Autodesk Fusion 360 part; units mm, degrees
(part 2 of 2)
sketch "Sketch26" plane through (0, 0, -20) normal (0, 0, -1) x (1, 0, 0)
  line L0 (49.5, -31.5) -> (-49.5, 31.5) construction
  line L1 (-49.5, -31.5) -> (49.5, 31.5) construction
  line L2 (-46.9725, 28.9725) -> (-52.0275, 28.9725)
  line L3 (-52.0275, 28.9725) -> (-52.0275, 34.0275)
  line L4 (-52.0275, 34.0275) -> (-46.9725, 34.0275)
  line L5 (-46.9725, 34.0275) -> (-46.9725, 28.9725)
  line L6 (-46.9725, 28.9725) -> (-52.0275, 34.0275) construction
  line L7 (-52.0275, 28.9725) -> (-46.9725, 34.0275) construction
  line L8 (-37.9725, 28.9725) -> (-43.0275, 28.9725)
  line L9 (-43.0275, 28.9725) -> (-43.0275, 34.0275)
  line L10 (-43.0275, 34.0275) -> (-37.9725, 34.0275)
  line L11 (-37.9725, 34.0275) -> (-37.9725, 28.9725)
  line L12 (-28.9725, 28.9725) -> (-34.0275, 28.9725)
  line L13 (-34.0275, 28.9725) -> (-34.0275, 34.0275)
  line L14 (-34.0275, 34.0275) -> (-28.9725, 34.0275)
  line L15 (-28.9725, 34.0275) -> (-28.9725, 28.9725)
  line L16 (-19.9725, 28.9725) -> (-25.0275, 28.9725)
  line L17 (-25.0275, 28.9725) -> (-25.0275, 34.0275)
  line L18 (-25.0275, 34.0275) -> (-19.9725, 34.0275)
  line L19 (-19.9725, 34.0275) -> (-19.9725, 28.9725)
  line L20 (-10.9725, 28.9725) -> (-16.0275, 28.9725)
  line L21 (-16.0275, 28.9725) -> (-16.0275, 34.0275)
  line L22 (-16.0275, 34.0275) -> (-10.9725, 34.0275)
  line L23 (-10.9725, 34.0275) -> (-10.9725, 28.9725)
  line L24 (-1.9725, 28.9725) -> (-7.0275, 28.9725)
  line L25 (-7.0275, 28.9725) -> (-7.0275, 34.0275)
  line L26 (-7.0275, 34.0275) -> (-1.9725, 34.0275)
  line L27 (-1.9725, 34.0275) -> (-1.9725, 28.9725)
  line L28 (7.0275, 28.9725) -> (1.9725, 28.9725)
  line L29 (1.9725, 28.9725) -> (1.9725, 34.0275)
  line L30 (1.9725, 34.0275) -> (7.0275, 34.0275)
  line L31 (7.0275, 34.0275) -> (7.0275, 28.9725)
  line L32 (16.0275, 28.9725) -> (10.9725, 28.9725)
  line L33 (10.9725, 28.9725) -> (10.9725, 34.0275)
  line L34 (10.9725, 34.0275) -> (16.0275, 34.0275)
  line L35 (16.0275, 34.0275) -> (16.0275, 28.9725)
  line L36 (25.0275, 28.9725) -> (19.9725, 28.9725)
  line L37 (19.9725, 28.9725) -> (19.9725, 34.0275)
  line L38 (19.9725, 34.0275) -> (25.0275, 34.0275)
  line L39 (25.0275, 34.0275) -> (25.0275, 28.9725)
  line L40 (34.0275, 28.9725) -> (28.9725, 28.9725)
  line L41 (28.9725, 28.9725) -> (28.9725, 34.0275)
  line L42 (28.9725, 34.0275) -> (34.0275, 34.0275)
  line L43 (34.0275, 34.0275) -> (34.0275, 28.9725)
  line L44 (43.0275, 28.9725) -> (37.9725, 28.9725)
  line L45 (37.9725, 28.9725) -> (37.9725, 34.0275)
  line L46 (37.9725, 34.0275) -> (43.0275, 34.0275)
  line L47 (43.0275, 34.0275) -> (43.0275, 28.9725)
  line L48 (52.0275, 28.9725) -> (46.9725, 28.9725)
  line L49 (46.9725, 28.9725) -> (46.9725, 34.0275)
  line L50 (46.9725, 34.0275) -> (52.0275, 34.0275)
  line L51 (52.0275, 34.0275) -> (52.0275, 28.9725)
  line L52 (-46.9725, 19.9725) -> (-52.0275, 19.9725)
  line L53 (-52.0275, 19.9725) -> (-52.0275, 25.0275)
  line L54 (-52.0275, 25.0275) -> (-46.9725, 25.0275)
  line L55 (-46.9725, 25.0275) -> (-46.9725, 19.9725)
  line L56 (-37.9725, 19.9725) -> (-43.0275, 19.9725)
  line L57 (-43.0275, 19.9725) -> (-43.0275, 25.0275)
  line L58 (-43.0275, 25.0275) -> (-37.9725, 25.0275)
  line L59 (-37.9725, 25.0275) -> (-37.9725, 19.9725)
  line L60 (-28.9725, 19.9725) -> (-34.0275, 19.9725)
  line L61 (-34.0275, 19.9725) -> (-34.0275, 25.0275)
  line L62 (-34.0275, 25.0275) -> (-28.9725, 25.0275)
  line L63 (-28.9725, 25.0275) -> (-28.9725, 19.9725)
  line L64 (-19.9725, 19.9725) -> (-25.0275, 19.9725)
  line L65 (-25.0275, 19.9725) -> (-25.0275, 25.0275)
  line L66 (-25.0275, 25.0275) -> (-19.9725, 25.0275)
  line L67 (-19.9725, 25.0275) -> (-19.9725, 19.9725)
  line L68 (-10.9725, 19.9725) -> (-16.0275, 19.9725)
  line L69 (-16.0275, 19.9725) -> (-16.0275, 25.0275)
  line L70 (-16.0275, 25.0275) -> (-10.9725, 25.0275)
  line L71 (-10.9725, 25.0275) -> (-10.9725, 19.9725)
  line L72 (-1.9725, 19.9725) -> (-7.0275, 19.9725)
  line L73 (-7.0275, 19.9725) -> (-7.0275, 25.0275)
  line L74 (-7.0275, 25.0275) -> (-1.9725, 25.0275)
  line L75 (-1.9725, 25.0275) -> (-1.9725, 19.9725)
  line L76 (7.0275, 19.9725) -> (1.9725, 19.9725)
  line L77 (1.9725, 19.9725) -> (1.9725, 25.0275)
  line L78 (1.9725, 25.0275) -> (7.0275, 25.0275)
  line L79 (7.0275, 25.0275) -> (7.0275, 19.9725)
  line L80 (16.0275, 19.9725) -> (10.9725, 19.9725)
  line L81 (10.9725, 19.9725) -> (10.9725, 25.0275)
  line L82 (10.9725, 25.0275) -> (16.0275, 25.0275)
  line L83 (16.0275, 25.0275) -> (16.0275, 19.9725)
  line L84 (25.0275, 19.9725) -> (19.9725, 19.9725)
  line L85 (19.9725, 19.9725) -> (19.9725, 25.0275)
  line L86 (19.9725, 25.0275) -> (25.0275, 25.0275)
  line L87 (25.0275, 25.0275) -> (25.0275, 19.9725)
  line L88 (34.0275, 19.9725) -> (28.9725, 19.9725)
  line L89 (28.9725, 19.9725) -> (28.9725, 25.0275)
  line L90 (28.9725, 25.0275) -> (34.0275, 25.0275)
  line L91 (34.0275, 25.0275) -> (34.0275, 19.9725)
  line L92 (43.0275, 19.9725) -> (37.9725, 19.9725)
  line L93 (37.9725, 19.9725) -> (37.9725, 25.0275)
  line L94 (37.9725, 25.0275) -> (43.0275, 25.0275)
  line L95 (43.0275, 25.0275) -> (43.0275, 19.9725)
  line L96 (52.0275, 19.9725) -> (46.9725, 19.9725)
  line L97 (46.9725, 19.9725) -> (46.9725, 25.0275)
  line L98 (46.9725, 25.0275) -> (52.0275, 25.0275)
  line L99 (52.0275, 25.0275) -> (52.0275, 19.9725)
  line L100 (-46.9725, 10.9725) -> (-52.0275, 10.9725)
  line L101 (-52.0275, 10.9725) -> (-52.0275, 16.0275)
  line L102 (-52.0275, 16.0275) -> (-46.9725, 16.0275)
  line L103 (-46.9725, 16.0275) -> (-46.9725, 10.9725)
  line L104 (-37.9725, 10.9725) -> (-43.0275, 10.9725)
  line L105 (-43.0275, 10.9725) -> (-43.0275, 16.0275)
  line L106 (-43.0275, 16.0275) -> (-37.9725, 16.0275)
  line L107 (-37.9725, 16.0275) -> (-37.9725, 10.9725)
  line L108 (-28.9725, 10.9725) -> (-34.0275, 10.9725)
  line L109 (-34.0275, 10.9725) -> (-34.0275, 16.0275)
  line L110 (-34.0275, 16.0275) -> (-28.9725, 16.0275)
  line L111 (-28.9725, 16.0275) -> (-28.9725, 10.9725)
  line L112 (-19.9725, 10.9725) -> (-25.0275, 10.9725)
  line L113 (-25.0275, 10.9725) -> (-25.0275, 16.0275)
  line L114 (-25.0275, 16.0275) -> (-19.9725, 16.0275)
  line L115 (-19.9725, 16.0275) -> (-19.9725, 10.9725)
  line L116 (-10.9725, 10.9725) -> (-16.0275, 10.9725)
  line L117 (-16.0275, 10.9725) -> (-16.0275, 16.0275)
  line L118 (-16.0275, 16.0275) -> (-10.9725, 16.0275)
  line L119 (-10.9725, 16.0275) -> (-10.9725, 10.9725)
  line L120 (-1.9725, 10.9725) -> (-7.0275, 10.9725)
  line L121 (-7.0275, 10.9725) -> (-7.0275, 16.0275)
  line L122 (-7.0275, 16.0275) -> (-1.9725, 16.0275)
  line L123 (-1.9725, 16.0275) -> (-1.9725, 10.9725)
  line L124 (7.0275, 10.9725) -> (1.9725, 10.9725)
  line L125 (1.9725, 10.9725) -> (1.9725, 16.0275)
  line L126 (1.9725, 16.0275) -> (7.0275, 16.0275)
  line L127 (7.0275, 16.0275) -> (7.0275, 10.9725)
  line L128 (16.0275, 10.9725) -> (10.9725, 10.9725)
  line L129 (10.9725, 10.9725) -> (10.9725, 16.0275)
  line L130 (10.9725, 16.0275) -> (16.0275, 16.0275)
  line L131 (16.0275, 16.0275) -> (16.0275, 10.9725)
  line L132 (25.0275, 10.9725) -> (19.9725, 10.9725)
  line L133 (19.9725, 10.9725) -> (19.9725, 16.0275)
  line L134 (19.9725, 16.0275) -> (25.0275, 16.0275)
  line L135 (25.0275, 16.0275) -> (25.0275, 10.9725)
  line L136 (34.0275, 10.9725) -> (28.9725, 10.9725)
  line L137 (28.9725, 10.9725) -> (28.9725, 16.0275)
  line L138 (28.9725, 16.0275) -> (34.0275, 16.0275)
  line L139 (34.0275, 16.0275) -> (34.0275, 10.9725)
  line L140 (43.0275, 10.9725) -> (37.9725, 10.9725)
  line L141 (37.9725, 10.9725) -> (37.9725, 16.0275)
  line L142 (37.9725, 16.0275) -> (43.0275, 16.0275)
  line L143 (43.0275, 16.0275) -> (43.0275, 10.9725)
  line L144 (52.0275, 10.9725) -> (46.9725, 10.9725)
  line L145 (46.9725, 10.9725) -> (46.9725, 16.0275)
  line L146 (46.9725, 16.0275) -> (52.0275, 16.0275)
  line L147 (52.0275, 16.0275) -> (52.0275, 10.9725)
  line L148 (-46.9725, 1.9725) -> (-52.0275, 1.9725)
  line L149 (-52.0275, 1.9725) -> (-52.0275, 7.0275)
  line L150 (-52.0275, 7.0275) -> (-46.9725, 7.0275)
  line L151 (-46.9725, 7.0275) -> (-46.9725, 1.9725)
  line L152 (-37.9725, 1.9725) -> (-43.0275, 1.9725)
  line L153 (-43.0275, 1.9725) -> (-43.0275, 7.0275)
  line L154 (-43.0275, 7.0275) -> (-37.9725, 7.0275)
  line L155 (-37.9725, 7.0275) -> (-37.9725, 1.9725)
  line L156 (-28.9725, 1.9725) -> (-34.0275, 1.9725)
  line L157 (-34.0275, 1.9725) -> (-34.0275, 7.0275)
  line L158 (-34.0275, 7.0275) -> (-28.9725, 7.0275)
  line L159 (-28.9725, 7.0275) -> (-28.9725, 1.9725)
  line L160 (-19.9725, 1.9725) -> (-25.0275, 1.9725)
  line L161 (-25.0275, 1.9725) -> (-25.0275, 7.0275)
  line L162 (-25.0275, 7.0275) -> (-19.9725, 7.0275)
  line L163 (-19.9725, 7.0275) -> (-19.9725, 1.9725)
  line L164 (-10.9725, 1.9725) -> (-16.0275, 1.9725)
  line L165 (-16.0275, 1.9725) -> (-16.0275, 7.0275)
  line L166 (-16.0275, 7.0275) -> (-10.9725, 7.0275)
  line L167 (-10.9725, 7.0275) -> (-10.9725, 1.9725)
  line L168 (-1.9725, 1.9725) -> (-7.0275, 1.9725)
  line L169 (-7.0275, 1.9725) -> (-7.0275, 7.0275)
  line L170 (-7.0275, 7.0275) -> (-1.9725, 7.0275)
  line L171 (-1.9725, 7.0275) -> (-1.9725, 1.9725)
  line L172 (7.0275, 1.9725) -> (1.9725, 1.9725)
  line L173 (1.9725, 1.9725) -> (1.9725, 7.0275)
  line L174 (1.9725, 7.0275) -> (7.0275, 7.0275)
  line L175 (7.0275, 7.0275) -> (7.0275, 1.9725)
  line L176 (16.0275, 1.9725) -> (10.9725, 1.9725)
  line L177 (10.9725, 1.9725) -> (10.9725, 7.0275)
  line L178 (10.9725, 7.0275) -> (16.0275, 7.0275)
  line L179 (16.0275, 7.0275) -> (16.0275, 1.9725)
  line L180 (25.0275, 1.9725) -> (19.9725, 1.9725)
  line L181 (19.9725, 1.9725) -> (19.9725, 7.0275)
  line L182 (19.9725, 7.0275) -> (25.0275, 7.0275)
  line L183 (25.0275, 7.0275) -> (25.0275, 1.9725)
  line L184 (34.0275, 1.9725) -> (28.9725, 1.9725)
  line L185 (28.9725, 1.9725) -> (28.9725, 7.0275)
  line L186 (28.9725, 7.0275) -> (34.0275, 7.0275)
  line L187 (34.0275, 7.0275) -> (34.0275, 1.9725)
  line L188 (43.0275, 1.9725) -> (37.9725, 1.9725)
  line L189 (37.9725, 1.9725) -> (37.9725, 7.0275)
  line L190 (37.9725, 7.0275) -> (43.0275, 7.0275)
  line L191 (43.0275, 7.0275) -> (43.0275, 1.9725)
  line L192 (52.0275, 1.9725) -> (46.9725, 1.9725)
  line L193 (46.9725, 1.9725) -> (46.9725, 7.0275)
  line L194 (46.9725, 7.0275) -> (52.0275, 7.0275)
  line L195 (52.0275, 7.0275) -> (52.0275, 1.9725)
  line L196 (-46.9725, -7.0275) -> (-52.0275, -7.0275)
  line L197 (-52.0275, -7.0275) -> (-52.0275, -1.9725)
  line L198 (-52.0275, -1.9725) -> (-46.9725, -1.9725)
  line L199 (-46.9725, -1.9725) -> (-46.9725, -7.0275)
  line L200 (-37.9725, -7.0275) -> (-43.0275, -7.0275)
  line L201 (-43.0275, -7.0275) -> (-43.0275, -1.9725)
  line L202 (-43.0275, -1.9725) -> (-37.9725, -1.9725)
  line L203 (-37.9725, -1.9725) -> (-37.9725, -7.0275)
  line L204 (-28.9725, -7.0275) -> (-34.0275, -7.0275)
  line L205 (-34.0275, -7.0275) -> (-34.0275, -1.9725)
  line L206 (-34.0275, -1.9725) -> (-28.9725, -1.9725)
  line L207 (-28.9725, -1.9725) -> (-28.9725, -7.0275)
  line L208 (-19.9725, -7.0275) -> (-25.0275, -7.0275)
  line L209 (-25.0275, -7.0275) -> (-25.0275, -1.9725)
  line L210 (-25.0275, -1.9725) -> (-19.9725, -1.9725)
  line L211 (-19.9725, -1.9725) -> (-19.9725, -7.0275)
  line L212 (-10.9725, -7.0275) -> (-16.0275, -7.0275)
  line L213 (-16.0275, -7.0275) -> (-16.0275, -1.9725)
  line L214 (-16.0275, -1.9725) -> (-10.9725, -1.9725)
  line L215 (-10.9725, -1.9725) -> (-10.9725, -7.0275)
  line L216 (-1.9725, -7.0275) -> (-7.0275, -7.0275)
  line L217 (-7.0275, -7.0275) -> (-7.0275, -1.9725)
  line L218 (-7.0275, -1.9725) -> (-1.9725, -1.9725)
  line L219 (-1.9725, -1.9725) -> (-1.9725, -7.0275)
  line L220 (7.0275, -7.0275) -> (1.9725, -7.0275)
  line L221 (1.9725, -7.0275) -> (1.9725, -1.9725)
  line L222 (1.9725, -1.9725) -> (7.0275, -1.9725)
  line L223 (7.0275, -1.9725) -> (7.0275, -7.0275)
  line L224 (16.0275, -7.0275) -> (10.9725, -7.0275)
  line L225 (10.9725, -7.0275) -> (10.9725, -1.9725)
  line L226 (10.9725, -1.9725) -> (16.0275, -1.9725)
  line L227 (16.0275, -1.9725) -> (16.0275, -7.0275)
  line L228 (25.0275, -7.0275) -> (19.9725, -7.0275)
  line L229 (19.9725, -7.0275) -> (19.9725, -1.9725)
  line L230 (19.9725, -1.9725) -> (25.0275, -1.9725)
  line L231 (25.0275, -1.9725) -> (25.0275, -7.0275)
  line L232 (34.0275, -7.0275) -> (28.9725, -7.0275)
  line L233 (28.9725, -7.0275) -> (28.9725, -1.9725)
  line L234 (28.9725, -1.9725) -> (34.0275, -1.9725)
  line L235 (34.0275, -1.9725) -> (34.0275, -7.0275)
  line L236 (43.0275, -7.0275) -> (37.9725, -7.0275)
  line L237 (37.9725, -7.0275) -> (37.9725, -1.9725)
  line L238 (37.9725, -1.9725) -> (43.0275, -1.9725)
  line L239 (43.0275, -1.9725) -> (43.0275, -7.0275)
  line L240 (52.0275, -7.0275) -> (46.9725, -7.0275)
  line L241 (46.9725, -7.0275) -> (46.9725, -1.9725)
  line L242 (46.9725, -1.9725) -> (52.0275, -1.9725)
  line L243 (52.0275, -1.9725) -> (52.0275, -7.0275)
  line L244 (-46.9725, -16.0275) -> (-52.0275, -16.0275)
  line L245 (-52.0275, -16.0275) -> (-52.0275, -10.9725)
  line L246 (-52.0275, -10.9725) -> (-46.9725, -10.9725)
  line L247 (-46.9725, -10.9725) -> (-46.9725, -16.0275)
  line L248 (-37.9725, -16.0275) -> (-43.0275, -16.0275)
  line L249 (-43.0275, -16.0275) -> (-43.0275, -10.9725)
  line L250 (-43.0275, -10.9725) -> (-37.9725, -10.9725)
  line L251 (-37.9725, -10.9725) -> (-37.9725, -16.0275)
  line L252 (-28.9725, -16.0275) -> (-34.0275, -16.0275)
  line L253 (-34.0275, -16.0275) -> (-34.0275, -10.9725)
  line L254 (-34.0275, -10.9725) -> (-28.9725, -10.9725)
  line L255 (-28.9725, -10.9725) -> (-28.9725, -16.0275)
  line L256 (-19.9725, -16.0275) -> (-25.0275, -16.0275)
  line L257 (-25.0275, -16.0275) -> (-25.0275, -10.9725)
  line L258 (-25.0275, -10.9725) -> (-19.9725, -10.9725)
  line L259 (-19.9725, -10.9725) -> (-19.9725, -16.0275)
  line L260 (-10.9725, -16.0275) -> (-16.0275, -16.0275)
  line L261 (-16.0275, -16.0275) -> (-16.0275, -10.9725)
  line L262 (-16.0275, -10.9725) -> (-10.9725, -10.9725)
  line L263 (-10.9725, -10.9725) -> (-10.9725, -16.0275)
  line L264 (-1.9725, -16.0275) -> (-7.0275, -16.0275)
  line L265 (-7.0275, -16.0275) -> (-7.0275, -10.9725)
  line L266 (-7.0275, -10.9725) -> (-1.9725, -10.9725)
  line L267 (-1.9725, -10.9725) -> (-1.9725, -16.0275)
  line L268 (7.0275, -16.0275) -> (1.9725, -16.0275)
  line L269 (1.9725, -16.0275) -> (1.9725, -10.9725)
  line L270 (1.9725, -10.9725) -> (7.0275, -10.9725)
  line L271 (7.0275, -10.9725) -> (7.0275, -16.0275)
  line L272 (16.0275, -16.0275) -> (10.9725, -16.0275)
  line L273 (10.9725, -16.0275) -> (10.9725, -10.9725)
  line L274 (10.9725, -10.9725) -> (16.0275, -10.9725)
  line L275 (16.0275, -10.9725) -> (16.0275, -16.0275)
  line L276 (25.0275, -16.0275) -> (19.9725, -16.0275)
  line L277 (19.9725, -16.0275) -> (19.9725, -10.9725)
  line L278 (19.9725, -10.9725) -> (25.0275, -10.9725)
  line L279 (25.0275, -10.9725) -> (25.0275, -16.0275)
  line L280 (34.0275, -16.0275) -> (28.9725, -16.0275)
  line L281 (28.9725, -16.0275) -> (28.9725, -10.9725)
  line L282 (28.9725, -10.9725) -> (34.0275, -10.9725)
  line L283 (34.0275, -10.9725) -> (34.0275, -16.0275)
  line L284 (43.0275, -16.0275) -> (37.9725, -16.0275)
  line L285 (37.9725, -16.0275) -> (37.9725, -10.9725)
  line L286 (37.9725, -10.9725) -> (43.0275, -10.9725)
  line L287 (43.0275, -10.9725) -> (43.0275, -16.0275)
  line L288 (52.0275, -16.0275) -> (46.9725, -16.0275)
  line L289 (46.9725, -16.0275) -> (46.9725, -10.9725)
  line L290 (46.9725, -10.9725) -> (52.0275, -10.9725)
  line L291 (52.0275, -10.9725) -> (52.0275, -16.0275)
  line L292 (-46.9725, -25.0275) -> (-52.0275, -25.0275)
  line L293 (-52.0275, -25.0275) -> (-52.0275, -19.9725)
  line L294 (-52.0275, -19.9725) -> (-46.9725, -19.9725)
  line L295 (-46.9725, -19.9725) -> (-46.9725, -25.0275)
  line L296 (-37.9725, -25.0275) -> (-43.0275, -25.0275)
  line L297 (-43.0275, -25.0275) -> (-43.0275, -19.9725)
  line L298 (-43.0275, -19.9725) -> (-37.9725, -19.9725)
  line L299 (-37.9725, -19.9725) -> (-37.9725, -25.0275)
  line L300 (-28.9725, -25.0275) -> (-34.0275, -25.0275)
  line L301 (-34.0275, -25.0275) -> (-34.0275, -19.9725)
  line L302 (-34.0275, -19.9725) -> (-28.9725, -19.9725)
  line L303 (-28.9725, -19.9725) -> (-28.9725, -25.0275)
  line L304 (-19.9725, -25.0275) -> (-25.0275, -25.0275)
  line L305 (-25.0275, -25.0275) -> (-25.0275, -19.9725)
  line L306 (-25.0275, -19.9725) -> (-19.9725, -19.9725)
  line L307 (-19.9725, -19.9725) -> (-19.9725, -25.0275)
  line L308 (-10.9725, -25.0275) -> (-16.0275, -25.0275)
  line L309 (-16.0275, -25.0275) -> (-16.0275, -19.9725)
  line L310 (-16.0275, -19.9725) -> (-10.9725, -19.9725)
  line L311 (-10.9725, -19.9725) -> (-10.9725, -25.0275)
  line L312 (-1.9725, -25.0275) -> (-7.0275, -25.0275)
  line L313 (-7.0275, -25.0275) -> (-7.0275, -19.9725)
  line L314 (-7.0275, -19.9725) -> (-1.9725, -19.9725)
  line L315 (-1.9725, -19.9725) -> (-1.9725, -25.0275)
  line L316 (7.0275, -25.0275) -> (1.9725, -25.0275)
  line L317 (1.9725, -25.0275) -> (1.9725, -19.9725)
  line L318 (1.9725, -19.9725) -> (7.0275, -19.9725)
  line L319 (7.0275, -19.9725) -> (7.0275, -25.0275)
  line L320 (16.0275, -25.0275) -> (10.9725, -25.0275)
  line L321 (10.9725, -25.0275) -> (10.9725, -19.9725)
  line L322 (10.9725, -19.9725) -> (16.0275, -19.9725)
  line L323 (16.0275, -19.9725) -> (16.0275, -25.0275)
  line L324 (25.0275, -25.0275) -> (19.9725, -25.0275)
  line L325 (19.9725, -25.0275) -> (19.9725, -19.9725)
  line L326 (19.9725, -19.9725) -> (25.0275, -19.9725)
  line L327 (25.0275, -19.9725) -> (25.0275, -25.0275)
  line L328 (34.0275, -25.0275) -> (28.9725, -25.0275)
  line L329 (28.9725, -25.0275) -> (28.9725, -19.9725)
  line L330 (28.9725, -19.9725) -> (34.0275, -19.9725)
  line L331 (34.0275, -19.9725) -> (34.0275, -25.0275)
  line L332 (43.0275, -25.0275) -> (37.9725, -25.0275)
  line L333 (37.9725, -25.0275) -> (37.9725, -19.9725)
  line L334 (37.9725, -19.9725) -> (43.0275, -19.9725)
  line L335 (43.0275, -19.9725) -> (43.0275, -25.0275)
  line L336 (52.0275, -25.0275) -> (46.9725, -25.0275)
  line L337 (46.9725, -25.0275) -> (46.9725, -19.9725)
  line L338 (46.9725, -19.9725) -> (52.0275, -19.9725)
  line L339 (52.0275, -19.9725) -> (52.0275, -25.0275)
  line L340 (-46.9725, -34.0275) -> (-52.0275, -34.0275)
  line L341 (-52.0275, -34.0275) -> (-52.0275, -28.9725)
  line L342 (-52.0275, -28.9725) -> (-46.9725, -28.9725)
  line L343 (-46.9725, -28.9725) -> (-46.9725, -34.0275)
  line L344 (-37.9725, -34.0275) -> (-43.0275, -34.0275)
  line L345 (-43.0275, -34.0275) -> (-43.0275, -28.9725)
  line L346 (-43.0275, -28.9725) -> (-37.9725, -28.9725)
  line L347 (-37.9725, -28.9725) -> (-37.9725, -34.0275)
  line L348 (-28.9725, -34.0275) -> (-34.0275, -34.0275)
  line L349 (-34.0275, -34.0275) -> (-34.0275, -28.9725)
  line L350 (-34.0275, -28.9725) -> (-28.9725, -28.9725)
  line L351 (-28.9725, -28.9725) -> (-28.9725, -34.0275)
  line L352 (-19.9725, -34.0275) -> (-25.0275, -34.0275)
  line L353 (-25.0275, -34.0275) -> (-25.0275, -28.9725)
  line L354 (-25.0275, -28.9725) -> (-19.9725, -28.9725)
  line L355 (-19.9725, -28.9725) -> (-19.9725, -34.0275)
  line L356 (-10.9725, -34.0275) -> (-16.0275, -34.0275)
  line L357 (-16.0275, -34.0275) -> (-16.0275, -28.9725)
  line L358 (-16.0275, -28.9725) -> (-10.9725, -28.9725)
  line L359 (-10.9725, -28.9725) -> (-10.9725, -34.0275)
  line L360 (-1.9725, -34.0275) -> (-7.0275, -34.0275)
  line L361 (-7.0275, -34.0275) -> (-7.0275, -28.9725)
  line L362 (-7.0275, -28.9725) -> (-1.9725, -28.9725)
  line L363 (-1.9725, -28.9725) -> (-1.9725, -34.0275)
  line L364 (7.0275, -34.0275) -> (1.9725, -34.0275)
  line L365 (1.9725, -34.0275) -> (1.9725, -28.9725)
  line L366 (1.9725, -28.9725) -> (7.0275, -28.9725)
  line L367 (7.0275, -28.9725) -> (7.0275, -34.0275)
  line L368 (16.0275, -34.0275) -> (10.9725, -34.0275)
  line L369 (10.9725, -34.0275) -> (10.9725, -28.9725)
  line L370 (10.9725, -28.9725) -> (16.0275, -28.9725)
  line L371 (16.0275, -28.9725) -> (16.0275, -34.0275)
  line L372 (25.0275, -34.0275) -> (19.9725, -34.0275)
  line L373 (19.9725, -34.0275) -> (19.9725, -28.9725)
  line L374 (19.9725, -28.9725) -> (25.0275, -28.9725)
  line L375 (25.0275, -28.9725) -> (25.0275, -34.0275)
  line L376 (34.0275, -34.0275) -> (28.9725, -34.0275)
  line L377 (28.9725, -34.0275) -> (28.9725, -28.9725)
  line L378 (28.9725, -28.9725) -> (34.0275, -28.9725)
  line L379 (34.0275, -28.9725) -> (34.0275, -34.0275)
  line L380 (43.0275, -34.0275) -> (37.9725, -34.0275)
  line L381 (37.9725, -34.0275) -> (37.9725, -28.9725)
  line L382 (37.9725, -28.9725) -> (43.0275, -28.9725)
  line L383 (43.0275, -28.9725) -> (43.0275, -34.0275)
  line L384 (52.0275, -34.0275) -> (46.9725, -34.0275)
  line L385 (46.9725, -34.0275) -> (46.9725, -28.9725)
  line L386 (46.9725, -28.9725) -> (52.0275, -28.9725)
  line L387 (52.0275, -28.9725) -> (52.0275, -34.0275)
  point P0 (-49.5, 31.5)
  dimension "d252" = 99
  dimension "d253" = 63
  dimension "d254" = 5.055
  dimension "d255" = 5.055
  dimension "d258" = 99
  dimension "d259" = -63
  constraint coincident L0 origin
  constraint coincident L1 origin
  constraint perpendicular L2 L3
  constraint parallel L2 L4
  constraint parallel L3 L5
  constraint horizontal L2
  constraint coincident L6 P0
  constraint coincident L7 P0
  constraint coincident P0 L0.end
  measures "d252" distance of P0 L1.end
  measures "d253" distance of L1.start P0
  measures "d254" distance of L3.end L4.end
  measures "d255" distance of L2.end L3.end
extrude "Extrude28" cut sketch "Sketch26" against normal blind 10
ref_plane "WorkPlane28" through (0, 0, -20) normal (0, 0, -1) x (-1, 0, 0)
sketch "Sketch27" plane through (0, 0, -20) normal (0, 0, -1) x (1, 0, 0)
  line L0 (65.38, -44.37) -> (-65.38, -44.37)
  line L1 (-65.38, -44.37) -> (-65.38, 44.37)
  line L2 (-65.38, 44.37) -> (65.38, 44.37)
  line L3 (65.38, 44.37) -> (65.38, -44.37)
  line L4 (65.38, -44.37) -> (-65.38, 44.37) construction
  line L5 (-65.38, -44.37) -> (65.38, 44.37) construction
  line L6 (55.5275, -37.5275) -> (-55.5275, -37.5275)
  line L7 (-55.5275, -37.5275) -> (-55.5275, 37.5275)
  line L8 (-55.5275, 37.5275) -> (55.5275, 37.5275)
  line L9 (55.5275, 37.5275) -> (55.5275, -37.5275)
  line L10 (55.5275, -37.5275) -> (-55.5275, 37.5275) construction
  line L11 (-55.5275, -37.5275) -> (55.5275, 37.5275) construction
  dimension "d263" = 130.76
  dimension "d264" = 88.74
  dimension "d265" = 111.055
  dimension "d266" = 75.055
  constraint perpendicular L0 L1
  constraint parallel L0 L2
  constraint parallel L1 L3
  constraint horizontal L0
  constraint coincident L4 origin
  constraint coincident L5 origin
  constraint perpendicular L6 L7
  constraint parallel L6 L8
  constraint parallel L7 L9
  constraint horizontal L6
  constraint coincident L10 origin
  constraint coincident L11 origin
  measures "d263" distance of L1.end L2.end
  measures "d264" distance of L0.end L1.end
  measures "d265" distance of L7.end L8.end
  measures "d266" distance of L6.end L7.end
extrude "Extrude29" cut sketch "Sketch27" against normal blind 35
fillet "Fillet11" radius 5 4 edges at (-55.5275, -37.5275, -2.5) (-55.5275, 37.5275, -2.5) (55.5275, 37.5275, -2.5) (55.5275, -37.5275, -2.5)
fillet "Fillet12" radius 5 4 edges at (-65.38, -44.37, -2.5) (-65.38, 44.37, -2.5) (65.38, -44.37, -2.5) (65.38, 44.37, -2.5)
fillet "Fillet13" radius 5 4 edges at (68.38, -47.37, 0) (68.38, 47.37, 0) (-68.38, 47.37, 0) (-68.38, -47.37, 0)
ref_plane "WorkPlane29" through (0, 0, 20) normal (0, 0, 1) x (1, 0, 0)
sketch "Sketch28" plane through (0, 0, 20) normal (0, 0, 1) x (1, 0, 0)
ref_plane "WorkPlane30" through (0, 0, 20) normal (0, 0, 1) x (1, 0, 0)
sketch "Sketch29" plane through (0, 0, 20) normal (0, 0, 1) x (1, 0, 0)
  circle A0 centre (-53.38, 52.37) radius 3
  circle A1 centre (53.3798, 52.37) radius 3
  circle A2 centre (53.38, -52.37) radius 3
  circle A3 centre (-53.38, -52.37) radius 3
  dimension "d275" = 6
  dimension "d276" = 6
  dimension "d277" = 6
  dimension "d278" = 6
  measures "d275" diameter of A0
  measures "d276" diameter of A1
  measures "d277" diameter of A2
  measures "d278" diameter of A3
extrude "Extrude30" cut sketch "Sketch29" against normal blind 40
fillet "Fillet15" radius 2 16 edges at (-58.38, 47.37, 0) (-58.38, 57.37, 0) (48.38, 47.37, 0) (48.38, 57.37, 0) (58.38, 57.37, 0) (-48.38, 47.37, 0) (-48.38, 57.37, 0) (58.38, 47.37, 0) (58.38, -47.37, 0) (-48.38, -47.37, 0) (-48.38, -57.37, 0) (58.38, -57.37, 0) (48.38, -47.37, 0) (48.38, -57.37, 0) (-58.38, -47.37, 0) (-58.38, -57.37, 0)
ref_plane "WorkPlane31" through (0, -47.37, 0) normal (0, -1, 0) x (1, 0, 0)
sketch "Sketch34" plane through (68.38, 0, 0) normal (1, 0, 0) x (0, 1, 0)
  line L0 (42.37, -20) -> (42.37, 20)
  line L1 (42.37, 20) -> (-42.37, 20)
  line L2 (-42.37, 20) -> (-42.37, -20)
  line L3 (-42.37, -20) -> (42.37, -20)
  line L4 (-35, 15) -> (35, 15)
  line L5 (-35, 5) -> (35, 5)
  line L6 (-35, -5) -> (35, -5)
  line L7 (-35, -15) -> (35, -15)
  circle A0 centre (-35, -15) radius 3
  circle A1 centre (35, -15) radius 3
  circle A2 centre (-35, -5) radius 3
  circle A3 centre (35, -5) radius 3
  circle A4 centre (-35, 5) radius 3
  circle A5 centre (35, 5) radius 3
  circle A6 centre (-35, 15) radius 3
  circle A7 centre (35, 15) radius 3
  line L8 (35, 12) -> (-35, 12)
  line L9 (-35, 12) -> (-35, 18)
  line L10 (-35, 18) -> (35, 18)
  line L11 (35, 18) -> (35, 12)
  line L12 (35, 12) -> (-35, 18) construction
  line L13 (-35, 12) -> (35, 18) construction
  line L14 (35, 2) -> (-35, 2)
  line L15 (-35, 2) -> (-35, 8)
  line L16 (-35, 8) -> (35, 8)
  line L17 (35, 8) -> (35, 2)
  line L18 (35, 2) -> (-35, 8) construction
  line L19 (-35, 2) -> (35, 8) construction
  line L20 (35, -8) -> (-35, -8)
  line L21 (-35, -8) -> (-35, -2)
  line L22 (-35, -2) -> (35, -2)
  line L23 (35, -2) -> (35, -8)
  line L24 (35, -8) -> (-35, -2) construction
  line L25 (-35, -8) -> (35, -2) construction
  line L26 (35, -12) -> (-35, -12)
  line L27 (-35, -12) -> (-35, -18)
  line L28 (-35, -18) -> (35, -18)
  line L29 (35, -18) -> (35, -12)
  line L30 (35, -12) -> (-35, -18) construction
  line L31 (-35, -12) -> (35, -18) construction
  point P0 (0, 15)
  point P1 (0, 5)
  point P2 (0, -5)
  point P3 (0, -15)
  dimension "d326" = 6
  dimension "d327" = 6
  dimension "d328" = 6
  dimension "d329" = 6
  dimension "d330" = 6
  dimension "d331" = 6
  dimension "d332" = 6
  dimension "d333" = 6
  dimension "d334" = 70
  dimension "d335" = 70
  dimension "d336" = 6
  dimension "d337" = 6
  dimension "d338" = 70
  dimension "d339" = 6
  dimension "d340" = 70
  constraint perpendicular L2 L4
  constraint horizontal L5
  constraint horizontal L6
  constraint horizontal L7
  constraint coincident L7.start A0.centre
  constraint coincident L7.end A1.centre
  constraint coincident L6.start A2.centre
  constraint coincident L6.end A3.centre
  constraint coincident L5.start A4.centre
  constraint coincident L5.end A5.centre
  constraint coincident L4.start A6.centre
  constraint coincident L4.end A7.centre
  constraint perpendicular L8 L9
  constraint parallel L8 L10
  constraint parallel L9 L11
  constraint horizontal L8
  constraint coincident L12 P0
  constraint coincident L13 P0
  constraint midpoint L4 P0
  constraint perpendicular L14 L15
  constraint parallel L14 L16
  constraint parallel L15 L17
  constraint horizontal L14
  constraint coincident L18 P1
  constraint coincident L19 P1
  constraint midpoint L5 P1
  constraint perpendicular L20 L21
  constraint parallel L20 L22
  constraint parallel L21 L23
  constraint horizontal L20
  constraint coincident L24 P2
  constraint coincident L25 P2
  constraint midpoint L6 P2
  constraint perpendicular L26 L27
  constraint parallel L26 L28
  constraint parallel L27 L29
  constraint horizontal L26
  constraint coincident L30 P3
  constraint coincident L31 P3
  constraint midpoint L7 P3
  measures "d326" diameter of A0
  measures "d327" diameter of A1
  measures "d328" diameter of A2
  measures "d329" diameter of A3
  measures "d330" diameter of A4
  measures "d331" diameter of A5
  measures "d332" diameter of A6
  measures "d333" diameter of A7
  measures "d334" distance of L9.end L10.end
  measures "d335" distance of L15.end L16.end
  measures "d336" distance of L14.end L15.end
  measures "d337" distance of L20.end L21.end
  measures "d338" distance of L21.end L22.end
  measures "d339" distance of L26.end L27.end
  measures "d340" distance of L27.end L28.end
extrude "Extrude35" cut sketch "Sketch34" against normal blind 3 contours L4 A6 L9 | L4 A6 L9 | A6 L9 | L4 A6 A7 L10 | L4 A6 A7 L8 | L4 A7 L11 | L4 A7 L11 | A7 L11 | L5 A4 L15 | L5 A4 L15 | A4 L15 | L5 A4 A5 L16 | L5 A4 A5 L14 | L5 A5 L17 | L5 A5 L17 | A5 L17 | L6 A2 L21 | L6 A2 L21 | A2 L21 | L6 A2 A3 L22 | L6 A2 A3 L20 | L6 A3 L23 | L6 A3 L23 | A3 L23 | L7 A0 L27 | A0 L27 | L7 A0 L27 | L7 A0 A1 L26 | L7 A0 A1 L28 | L7 A1 L29 | L7 A1 L29 | A1 L29
sketch "Sketch35" plane through (-68.38, 0, 0) normal (-1, 0, 0) x (0, -1, 0)
  line L0 (42.37, -20) -> (42.37, 20)
  line L1 (42.37, 20) -> (-42.37, 20)
  line L2 (-42.37, 20) -> (-42.37, -20)
  line L3 (-42.37, -20) -> (42.37, -20)
  line L4 (-35, 15) -> (35, 15)
  line L5 (-35, 5) -> (35, 5)
  line L6 (-35, -5) -> (35, -5)
  line L7 (-35, -15) -> (35, -15)
  circle A0 centre (-35, 15) radius 3
  circle A1 centre (-35, 5) radius 3
  circle A2 centre (-35, -5) radius 3
  circle A3 centre (-35, -15) radius 3
  circle A4 centre (35, 15) radius 3
  circle A5 centre (35, 5) radius 3
  circle A6 centre (35, -5) radius 3
  circle A7 centre (35, -15) radius 3
  line L8 (35, 12) -> (-35, 12)
  line L9 (-35, 12) -> (-35, 18)
  line L10 (-35, 18) -> (35, 18)
  line L11 (35, 18) -> (35, 12)
  line L12 (35, 12) -> (-35, 18) construction
  line L13 (-35, 12) -> (35, 18) construction
  line L14 (35, 2) -> (-35, 2)
  line L15 (-35, 2) -> (-35, 8)
  line L16 (-35, 8) -> (35, 8)
  line L17 (35, 8) -> (35, 2)
  line L18 (35, 2) -> (-35, 8) construction
  line L19 (-35, 2) -> (35, 8) construction
  line L20 (35, -8) -> (-35, -8)
  line L21 (-35, -8) -> (-35, -2)
  line L22 (-35, -2) -> (35, -2)
  line L23 (35, -2) -> (35, -8)
  line L24 (35, -8) -> (-35, -2) construction
  line L25 (-35, -8) -> (35, -2) construction
  line L26 (35, -18) -> (-35, -18)
  line L27 (-35, -18) -> (-35, -12)
  line L28 (-35, -12) -> (35, -12)
  line L29 (35, -12) -> (35, -18)
  line L30 (35, -18) -> (-35, -12) construction
  line L31 (-35, -18) -> (35, -12) construction
  point P0 (0, 15)
  point P1 (0, 5)
  point P2 (0, -5)
  point P3 (0, -15)
  dimension "d343" = 6
  dimension "d344" = 6
  dimension "d345" = 6
  dimension "d346" = 6
  dimension "d347" = 6
  dimension "d348" = 6
  dimension "d349" = 6
  dimension "d350" = 6
  dimension "d351" = 70
  dimension "d352" = 6
  dimension "d353" = 70
  dimension "d354" = 6
  dimension "d355" = 70
  dimension "d356" = 6
  dimension "d357" = 6
  dimension "d358" = 70
  constraint horizontal L4
  constraint horizontal L5
  constraint horizontal L6
  constraint horizontal L7
  constraint coincident L4.start A0.centre
  constraint coincident L5.start A1.centre
  constraint coincident L6.start A2.centre
  constraint coincident L7.start A3.centre
  constraint coincident L4.end A4.centre
  constraint coincident L5.end A5.centre
  constraint coincident L6.end A6.centre
  constraint coincident L7.end A7.centre
  constraint perpendicular L8 L9
  constraint parallel L8 L10
  constraint parallel L9 L11
  constraint horizontal L8
  constraint coincident L12 P0
  constraint coincident L13 P0
  constraint midpoint L4 P0
  constraint perpendicular L14 L15
  constraint parallel L14 L16
  constraint parallel L15 L17
  constraint horizontal L14
  constraint coincident L18 P1
  constraint coincident L19 P1
  constraint midpoint L5 P1
  constraint perpendicular L20 L21
  constraint parallel L20 L22
  constraint parallel L21 L23
  constraint horizontal L20
  constraint coincident L24 P2
  constraint coincident L25 P2
  constraint midpoint L6 P2
  constraint perpendicular L26 L27
  constraint parallel L26 L28
  constraint parallel L27 L29
  constraint horizontal L26
  constraint coincident L30 P3
  constraint coincident L31 P3
  constraint midpoint L7 P3
  measures "d343" diameter of A0
  measures "d344" diameter of A1
  measures "d345" diameter of A2
  measures "d346" diameter of A3
  measures "d347" diameter of A4
  measures "d348" diameter of A5
  measures "d349" diameter of A6
  measures "d350" diameter of A7
  measures "d351" distance of L9.end L10.end
  measures "d352" distance of L8.end L9.end
  measures "d353" distance of L15.end L16.end
  measures "d354" distance of L14.end L15.end
  measures "d355" distance of L21.end L22.end
  measures "d356" distance of L20.end L21.end
  measures "d357" distance of L26.end L27.end
  measures "d358" distance of L27.end L28.end
extrude "Extrude36" cut sketch "Sketch35" against normal blind 3 contours L4 A0 L9 | L4 A0 L9 | A0 L9 | L4 A0 A4 L10 | L4 A0 A4 L8 | L4 A4 L11 | L4 A4 L11 | A4 L11 | L5 A1 L15 | L5 A1 L15 | A1 L15 | L5 A1 A5 L16 | L5 A1 A5 L14 | L5 A5 L17 | L5 A5 L17 | A5 L17 | L6 A2 L21 | L6 A2 L21 | A2 L21 | L6 A2 A6 L22 | L6 A2 A6 L20 | L6 A6 L23 | L6 A6 L23 | A6 L23 | L7 A3 L27 | L7 A3 L27 | A3 L27 | L7 A3 A7 L28 | L7 A3 A7 L26 | L7 A7 L29 | L7 A7 L29 | A7 L29
sketch "Sketch36" plane through (0, -47.37, 0) normal (0, -1, 0) x (1, 0, 0)
  line L0 (46.38, -20) -> (46.38, 20)
  line L1 (46.38, 20) -> (-46.38, 20)
  line L2 (-46.38, 20) -> (-46.38, -20)
  line L3 (-46.38, -20) -> (46.38, -20)
  line L4 (-40, 15) -> (40, 15)
  line L5 (-40, 5) -> (40, 5)
  line L6 (-40, -5) -> (40, -5)
  line L7 (-40, -15) -> (40, -15)
  circle A0 centre (-40, 15) radius 3
  circle A1 centre (40, 15) radius 3
  circle A2 centre (-40, 5) radius 3
  circle A3 centre (40, 5) radius 3
  circle A4 centre (-40, -5) radius 3
  circle A5 centre (40, -5) radius 3
  circle A6 centre (-40, -15) radius 3
  circle A7 centre (40, -15) radius 3
  line L8 (40, 12) -> (-40, 12)
  line L9 (-40, 12) -> (-40, 18)
  line L10 (-40, 18) -> (40, 18)
  line L11 (40, 18) -> (40, 12)
  line L12 (40, 12) -> (-40, 18) construction
  line L13 (-40, 12) -> (40, 18) construction
  line L14 (40, 2) -> (-40, 2)
  line L15 (-40, 2) -> (-40, 8)
  line L16 (-40, 8) -> (40, 8)
  line L17 (40, 8) -> (40, 2)
  line L18 (40, 2) -> (-40, 8) construction
  line L19 (-40, 2) -> (40, 8) construction
  line L20 (40, -8) -> (-40, -8)
  line L21 (-40, -8) -> (-40, -2)
  line L22 (-40, -2) -> (40, -2)
  line L23 (40, -2) -> (40, -8)
  line L24 (40, -8) -> (-40, -2) construction
  line L25 (-40, -8) -> (40, -2) construction
  line L26 (40, -18) -> (-40, -18)
  line L27 (-40, -18) -> (-40, -12)
  line L28 (-40, -12) -> (40, -12)
  line L29 (40, -12) -> (40, -18)
  line L30 (40, -18) -> (-40, -12) construction
  line L31 (-40, -18) -> (40, -12) construction
  point P0 (0, 15)
  point P1 (0, 5)
  point P2 (0, -5)
  point P3 (0, -15)
  dimension "d361" = 6
  dimension "d364" = 80
  dimension "d365" = -30
  dimension "d366" = 80
  dimension "d367" = 6
  dimension "d368" = 80
  dimension "d369" = 6
  dimension "d370" = 80
  dimension "d371" = 6
  dimension "d372" = 80
  dimension "d373" = 6
  constraint horizontal L4
  constraint horizontal L5
  constraint horizontal L6
  constraint horizontal L7
  constraint coincident L4.start A0.centre
  constraint perpendicular L8 L9
  constraint parallel L8 L10
  constraint parallel L9 L11
  constraint horizontal L8
  constraint coincident L12 P0
  constraint coincident L13 P0
  constraint midpoint L4 P0
  constraint perpendicular L14 L15
  constraint parallel L14 L16
  constraint parallel L15 L17
  constraint horizontal L14
  constraint coincident L18 P1
  constraint coincident L19 P1
  constraint midpoint L5 P1
  constraint perpendicular L20 L21
  constraint parallel L20 L22
  constraint parallel L21 L23
  constraint horizontal L20
  constraint coincident L24 P2
  constraint coincident L25 P2
  constraint midpoint L6 P2
  constraint perpendicular L26 L27
  constraint parallel L26 L28
  constraint parallel L27 L29
  constraint horizontal L26
  constraint coincident L30 P3
  constraint coincident L31 P3
  constraint midpoint L7 P3
  measures "d361" diameter of A0
  measures "d366" distance of L9.end L10.end
  measures "d367" distance of L8.end L9.end
  measures "d368" distance of L15.end L16.end
  measures "d369" distance of L14.end L15.end
  measures "d370" distance of L21.end L22.end
  measures "d371" distance of L20.end L21.end
  measures "d372" distance of L27.end L28.end
  measures "d373" distance of L26.end L27.end
extrude "Extrude37" cut sketch "Sketch36" against normal blind 3 contours L4 A0 L9 | L4 A0 L9 | A0 L9 | L4 A0 A1 L10 | L4 A0 A1 L8 | L4 A1 L11 | L4 A1 L11 | A1 L11 | L5 A2 L15 | L5 A2 L15 | A2 L15 | L5 A2 A3 L16 | L5 A2 A3 L14 | L5 A3 L17 | L5 A3 L17 | A3 L17 | L6 A4 L21 | L6 A4 L21 | A4 L21 | L6 A4 A5 L22 | L6 A4 A5 L20 | L6 A5 L23 | L6 A5 L23 | A5 L23 | L7 A6 L27 | L7 A6 L27 | A6 L27 | L7 A6 A7 L28 | L7 A6 A7 L26 | L7 A7 L29 | L7 A7 L29 | A7 L29
sketch "Sketch37" plane through (0, 47.37, 0) normal (0, 1, 0) x (-1, 0, 0)
  line L0 (46.38, -20) -> (46.38, 20)
  line L1 (46.38, 20) -> (-46.38, 20)
  line L2 (-46.38, 20) -> (-46.38, -20)
  line L3 (-46.38, -20) -> (46.38, -20)
  line L4 (-40, 15) -> (40, 15)
  circle A0 centre (-40, 15) radius 3
  circle A1 centre (40, 15) radius 3
  circle A2 centre (-40, 5) radius 3
  circle A3 centre (40, 5) radius 3
  circle A4 centre (-40, -5) radius 3
  circle A5 centre (40, -5) radius 3
  circle A6 centre (-40, -15) radius 3
  circle A7 centre (40, -15) radius 3
  line L5 (40, 12) -> (-40, 12)
  line L6 (-40, 12) -> (-40, 18)
  line L7 (-40, 18) -> (40, 18)
  line L8 (40, 18) -> (40, 12)
  line L9 (40, 12) -> (-40, 18) construction
  line L10 (-40, 12) -> (40, 18) construction
  line L11 (40, 2) -> (-40, 2)
  line L12 (-40, 2) -> (-40, 8)
  line L13 (-40, 8) -> (40, 8)
  line L14 (40, 8) -> (40, 2)
  line L15 (40, 2) -> (-40, 8) construction
  line L16 (-40, 2) -> (40, 8) construction
  line L17 (40, -8) -> (-40, -8)
  line L18 (-40, -8) -> (-40, -2)
  line L19 (-40, -2) -> (40, -2)
  line L20 (40, -2) -> (40, -8)
  line L21 (40, -8) -> (-40, -2) construction
  line L22 (-40, -8) -> (40, -2) construction
  line L23 (40, -18) -> (-40, -18)
  line L24 (-40, -18) -> (-40, -12)
  line L25 (-40, -12) -> (40, -12)
  line L26 (40, -12) -> (40, -18)
  line L27 (40, -18) -> (-40, -12) construction
  line L28 (-40, -18) -> (40, -12) construction
  point P0 (0, 15)
  point P1 (0, 5)
  point P2 (0, -5)
  point P3 (0, -15)
  dimension "d376" = 6
  dimension "d379" = 80
  dimension "d380" = -30
  dimension "d381" = 80
  dimension "d382" = 6
  dimension "d383" = 6
  dimension "d384" = 80
  dimension "d385" = 80
  dimension "d386" = 6
  dimension "d387" = 6
  dimension "d388" = 80
  constraint horizontal L4
  constraint coincident L4.start A0.centre
  constraint perpendicular L5 L6
  constraint parallel L5 L7
  constraint parallel L6 L8
  constraint horizontal L5
  constraint coincident L9 P0
  constraint coincident L10 P0
  constraint midpoint L4 P0
  constraint perpendicular L11 L12
  constraint parallel L11 L13
  constraint parallel L12 L14
  constraint horizontal L11
  constraint coincident L15 P1
  constraint coincident L16 P1
  constraint perpendicular L17 L18
  constraint parallel L17 L19
  constraint parallel L18 L20
  constraint horizontal L17
  constraint coincident L21 P2
  constraint coincident L22 P2
  constraint perpendicular L23 L24
  constraint parallel L23 L25
  constraint parallel L24 L26
  constraint horizontal L23
  constraint coincident L27 P3
  constraint coincident L28 P3
  measures "d376" diameter of A0
  measures "d381" distance of L6.end L7.end
  measures "d382" distance of L5.end L6.end
  measures "d383" distance of L11.end L12.end
  measures "d384" distance of L12.end L13.end
  measures "d385" distance of L18.end L19.end
  measures "d386" distance of L17.end L18.end
  measures "d387" distance of L23.end L24.end
  measures "d388" distance of L24.end L25.end
extrude "Extrude38" cut sketch "Sketch37" against normal blind 3 contours L4 A0 L6 | L4 A0 L6 | A0 L6 | L4 A0 A1 L7 | L4 A0 A1 L5 | L4 A1 L8 | L4 A1 L8 | A1 L8 | A2 L12 | A2 A3 L11 L13 | A2 L12 | A3 L14 | A3 L14 | A4 L18 | A4 A5 L17 L19 | A4 L18 | A5 L20 | A5 L20 | A6 L24 | A6 A7 L23 L25 | A6 L24 | A7 L26 | A7 L26
ref_plane "WorkPlane35" through (0, 0, -20) normal (0, 0, -1) x (-1, 0, 0)
